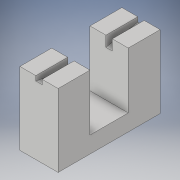
# Autodesk Inventor part: support
Saved by Autodesk Inventor 2018 (Build 220112000, 112)
## iProperties
Created: 2017-09-25
Part Number: support
Material: Generic
Document SubType Name: Modeling
Designer: ajay.john
Density: 1 g/cm^3
Appearance: Default
Author: ajay.john
Autodesk Inventor part; units mm, degrees
ref_plane "YZ Plane" through (0, 0, 0) normal (1, 0, 0) x (0, 1, 0)
ref_plane "XZ Plane" through (0, 0, 0) normal (0, 1, 0) x (-1, 0, 0)
ref_plane "XY Plane" through (0, 0, 0) normal (0, 0, 1) x (1, 0, 0)
sketch "Sketch1" plane through (0, 0, 0) normal (1, 0, 0) x (0, 1, 0)
  line L0 (0, 0) -> (114, 0)
  line L1 (114, 0) -> (114, -50)
  line L2 (0, -50) -> (114, -50)
  line L3 (0, -50) -> (0, 0)
  constraints: 8 end point, 2 perpendicular, 1 horizontal, 1 vertical
extrude "Extrusion1" add sketch "Sketch1" along normal blind 25
sketch "Sketch2" plane through (25, 0, 0) normal (1, 0, 0) x (0, 0, -1)
  line L0 (50, 114) -> (0, 114) projected
  line L1 (0, 114) -> (0, 79)
  line L2 (0, 114) -> (0, 0) projected
  line L3 (50, 0) -> (50, 114) projected
  line L4 (0, 79) -> (0, 106.71)
  line L5 (50, 79) -> (50, 97.46)
  line L6 (50, 97.46) -> (0, 106.71)
  line L7 (0, 0) -> (50, 0) projected
  line L8 (0, 106.71) -> (0, 0)
  line L9 (0, 0) -> (50, 0)
  line L10 (50, 0) -> (50, 97.46)
  constraints: 14 end point, 4 point on line, 2 collinear, 1 vertical
extrude "Extrusion2" add sketch "Sketch2" along normal blind 5 contours L3 L7 L2 L1 L6
mirror "Mirror1" about plane through (30, 51.2546, -24.2418) normal (1, 0, 0) of "Extrusion2", "Extrusion1"
sketch "Sketch3" plane through (0, 0, -50) normal (0, 0, -1) x (-1, 0, 0)
  line L0 (-60, 114) -> (-60, 0) projected
  line L1 (0, 0) -> (-60, 0) projected
  line L2 (-60, 0) -> (0, 0)
  line L3 (0, 0) -> (0, 25.8573)
  line L4 (0, 0) -> (0, 114) projected
  line L5 (-60, 25.8573) -> (0, 25.8573)
  line L6 (-60, 25.8573) -> (-60, 0)
  constraints: 8 end point, 2 perpendicular, 1 collinear, 1 point on line
extrude "Extrusion3" add sketch "Sketch3" along normal blind 30
mirror "Mirror2" about plane through (30, 12.9287, -80) normal (0, 0, -1) of "Extrusion2", "Extrusion1", "Mirror1", "Extrusion3"
body "Solid1"
